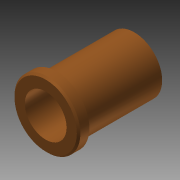
# Autodesk Inventor part: Tetrix Bronze Bushing (modified to fit vex couplers)
Saved by Autodesk Inventor 2014 SP1 (Build 180222100, 222)
## iProperties
Created: 2011-09-21
Part Number: Tetrix Bronze Bushing (modified to fit vex couplers)
Material: Bronze, Soft Tin
Document SubType Name: Modeling
Designer: MC
Density: 8.874 g/cm^3
Mass: 2.74755 g
Surface Area: 6.45814 cm^2
Volume: 0.309618 cm^3
Appearance: Bronze - Satin
Author: MC
Autodesk Inventor part; units mm, degrees
ref_plane "YZ Plane" through (0, 0, 0) normal (1, 0, 0) x (0, 1, 0)
ref_plane "XZ Plane" through (0, 0, 0) normal (0, 1, 0) x (-1, 0, 0)
ref_plane "XY Plane" through (0, 0, 0) normal (0, 0, 1) x (1, 0, 0)
sketch "Sketch1" plane through (0, 0, 0) normal (0, 0, 1) x (1, 0, 0)
  circle A0 centre (0, 0) radius 4.725
  circle A1 centre (0, 0) radius 3
  circle A2 centre (0, 0) radius 4
  dimension "d0" = 9.45
  dimension "d1" = 6
  dimension "d4" = 8
  constraints: 3 centre point, 3 coincident
  measures "d0" diameter of A0
  measures "d1" diameter of A1
  measures "d4" diameter of A2
extrude "Extrusion1" add sketch "Sketch1" along normal blind 1.55 contours A0 | A2
extrude "Extrusion2" add sketch "Sketch1" against normal blind 11.17 contours A2
chamfer "Chamfer1" distance 0.25 angle 45 1 edges at (-4.725, 0, 1.55)
body "Solid1"
